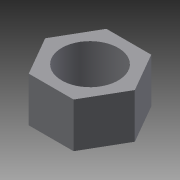
# Autodesk Inventor part: denso-gates-15 spacer
Saved by Autodesk Inventor 2015 (Build 190159000, 159)
## iProperties
Created: 2015-02-13
Part Number: denso-gates-15 spacer
Material: Generic
Document SubType Name: Modeling
Designer: robotics
Density: 1 g/cm^3
Appearance: Default
Author: robotics
Autodesk Inventor part; units mm, degrees
ref_plane "YZ Plane" through (0, 0, 0) normal (1, 0, 0) x (0, 1, 0)
ref_plane "XZ Plane" through (0, 0, 0) normal (0, 1, 0) x (-1, 0, 0)
ref_plane "XY Plane" through (0, 0, 0) normal (0, 0, 1) x (1, 0, 0)
sketch "Sketch1" plane through (0, 0, 0) normal (0, 1, 0) x (-1, 0, 0)
  circle A0 centre (0, 0) radius 6.4135 construction
  line L0 (-3.2067, 5.5543) -> (3.2068, 5.5543)
  line L1 (-3.2067, 5.5543) -> (-6.4135, 0)
  line L2 (-6.4135, 0) -> (-3.2068, -5.5543)
  line L3 (-3.2068, -5.5543) -> (3.2067, -5.5543)
  line L4 (3.2067, -5.5543) -> (6.4135, 0)
  line L5 (6.4135, 0) -> (3.2068, 5.5543)
  circle A1 centre (0, 0) radius 4.0386
  dimension "d0" = 12.827
  dimension "d1" = 8.0772
  constraints: 12 end point, 6 point on circle, 3 equal length, 2 centre point, 2 coincident, 2 horizontal, 2 parallel
  measures "d0" diameter of A0
  measures "d1" diameter of A1
extrude "Extrusion1" add sketch "Sketch1" along normal blind 6.4008
body "Solid1"
